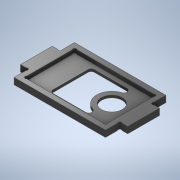
# Autodesk Inventor part: Trunk_servo_bottom_frame
Saved by Autodesk Inventor 2022 (Build 260153000, 153)
## iProperties
Part Number: Trunk_servo_bottom_frame
Material: アルミニウム 2014-T4
Document SubType Name: Sheet Metal
Designer: Masato Kubotera
Density: 2.8 g/cm^3
Appearance: 光沢 - 黒
Mass: 11.2606 g
Surface Area: 63.2089 cm^2
Volume: 7.90215 cm^3
Description: A2017 T4
Sheet Metal Rule: Default
Author: Masato Kubotera
Autodesk Inventor part; units mm, degrees
ref_plane "YZ Plane" through (0, 0, 0) normal (1, 0, 0) x (0, 1, 0)
ref_plane "XZ Plane" through (0, 0, 0) normal (0, 1, 0) x (-1, 0, 0)
ref_plane "XY Plane" through (0, 0, 0) normal (0, 0, 1) x (1, 0, 0)
sketch "スケッチ1" plane through (0, 0, 0) normal (0, 0, 1) x (1, 0, 0)
  line L0 (12, 16) -> (-29, 16) construction
  line L1 (-31, 14) -> (-31, -14) construction
  line L2 (-29, -16) -> (12, -16) construction
  line L3 (12, -16) -> (12, 16) construction
  line L4 (12, 16) -> (-31, -16) construction
  line L5 (-31, 16) -> (12, -16) construction
  line L6 (12, 0) -> (-31, 0) construction
  circle A0 centre (0, 0) radius 10.5 construction
  arc A1 (12, 10.583) -> (0, 16) centre (0, 0) ccw construction
  line L7 (-39.5, 14.4) -> (-39.5, -14.4) construction
  arc A2 (-29, 16) -> (-31, 14) centre (-29, 14) ccw construction
  arc A3 (-31, -14) -> (-29, -16) centre (-29, -14) ccw construction
  line L8 (-39.5, 14.4) -> (-30.9596, 14.4) construction
  line L9 (-39.5, -14.4) -> (-30.9596, -14.4) construction
  line L10 (-1, 13.5) -> (-28, 13.5) construction
  line L11 (-28, 13.5) -> (-28, -13.5) construction
  line L12 (-28, -13.5) -> (-1, -13.5) construction
  line L13 (-1, -13.5) -> (-1, 13.5) construction
  line L14 (-1, 13.5) -> (-28, -13.5) construction
  line L15 (-28, 13.5) -> (-1, -13.5) construction
  circle A4 centre (-1, 13.5) radius 1.35 construction
  circle A5 centre (-28, 13.5) radius 1.35 construction
  circle A6 centre (-1, -13.5) radius 1.35 construction
  circle A7 centre (-28, -13.5) radius 1.35 construction
  arc A8 (0, -16) -> (12, -10.583) centre (0, 0) ccw construction
  line L16 (11.9, 15.8) -> (11.9, 14.3151) construction
  line L17 (11.9, 15.8) -> (10.4151, 15.8) construction
  line L18 (-39.225, 15.8) -> (-39.225, 14.3151) construction
  arc A9 (-37.7401, 15.8) -> (-39.225, 14.3151) centre (-38.4825, 15.0575) ccw
  line L19 (11.9, -15.8) -> (10.4151, -15.8) construction
  arc A10 (-39.225, -14.3151) -> (-37.7401, -15.8) centre (-38.4825, -15.0575) ccw
  line L20 (-42.5, 19) -> (15, 19)
  line L21 (15, 19) -> (15, -19) construction
  line L22 (15, -19) -> (-42.5, -19)
  line L23 (-42.5, -19) -> (-42.5, 19) construction
  line L24 (-42.5, 19) -> (15, -19) construction
  line L25 (15, 19) -> (-42.5, -19) construction
  line L26 (15, 10) -> (16.4849, 10) construction
  line L27 (20, 10) -> (20, -10)
  line L28 (15, -10) -> (16.4849, -10) construction
  arc A11 (15, 11.4849) -> (16.4849, 10) centre (15.7425, 10.7425) ccw
  arc A12 (16.4849, -10) -> (15, -11.4849) centre (15.7425, -10.7425) ccw
  line L29 (-13.75, 19) -> (-13.75, -19) construction
  line L30 (15, 11.4849) -> (15, 19)
  line L31 (15, -11.4849) -> (15, -19)
  line L32 (-42.5, 10) -> (-43.9849, 10) construction
  line L33 (-47.5, 10) -> (-47.5, -10)
  line L34 (-42.5, -10) -> (-43.9849, -10) construction
  arc A13 (-43.9849, 10) -> (-42.5, 11.4849) centre (-43.2425, 10.7425) ccw
  arc A14 (-42.5, -11.4849) -> (-43.9849, -10) centre (-43.2425, -10.7425) ccw
  line L35 (-42.5, 11.4849) -> (-42.5, 19)
  line L36 (-42.5, -11.4849) -> (-42.5, -19)
  circle A15 centre (0, 0) radius 6 construction
  circle A16 centre (0, 0) radius 6.5
  line L37 (-3.5, 13) -> (-24, 13)
  line L38 (-26, 11) -> (-26, -11)
  line L39 (-3.5, -13) -> (-24, -13)
  arc A17 (-24, 13) -> (-26, 11) centre (-24, 11) ccw
  arc A18 (-26, -11) -> (-24, -13) centre (-24, -11) ccw
  line L40 (-1.5, 11) -> (-1.5, 10.9545)
  arc A19 (-2.8913, 9.0493) -> (-2.8913, -9.0493) centre (0, 0) ccw
  line L41 (-1.5, -10.9545) -> (-1.5, -11)
  arc A20 (-1.5, 11) -> (-3.5, 13) centre (-3.5, 11) ccw
  arc A21 (-3.5, -13) -> (-1.5, -11) centre (-3.5, -11) ccw
  arc A22 (-1.5, -10.9545) -> (-2.8913, -9.0493) centre (-3.5, -10.9545) ccw
  arc A23 (-2.8913, 9.0493) -> (-1.5, 10.9545) centre (-3.5, 10.9545) ccw
  arc A24 (11.9, 14.3151) -> (10.4151, 15.8) centre (11.1575, 15.0575) ccw
  arc A25 (10.4151, -15.8) -> (11.9, -14.3151) centre (11.1575, -15.0575) ccw
  line L42 (10.4151, 15.8) -> (-37.7401, 15.8)
  line L43 (11.9, 14.3151) -> (11.9, -14.3151)
  line L44 (10.4151, -15.8) -> (-37.7401, -15.8)
  line L45 (11.9, -14.3151) -> (11.9, -15.8) construction
  line L46 (-37.7401, -15.8) -> (-39.225, -15.8) construction
  line L47 (-39.225, -14.3151) -> (-39.225, -15.8) construction
  line L48 (-37.7401, 15.8) -> (-39.225, 15.8) construction
  line L49 (-39.225, 14.3151) -> (-39.225, -14.3151)
  line L50 (16.4849, 10) -> (20, 10)
  line L51 (16.4849, -10) -> (20, -10)
  line L52 (-43.9849, -10) -> (-47.5, -10)
  line L53 (-43.9849, 10) -> (-47.5, 10)
  point P0 (-9.5, 0)
  point P1 (-14.5, 0)
  point P2 (-13.75, 0)
  point P3 (-39.225, -14.3151)
  point P4 (-43.9849, -10)
  point P5 (-1.5, 13)
  point P6 (-26, 13)
  point P7 (-1.5, -13)
  point P8 (-26, -13)
  point P9 (-1.5, -13)
  point P10 (-1.5, 13)
  point P11 (-1.5, 9.3808)
  point P12 (-1.5, -9.3808)
  point P13 (11.9, -14.3151)
  point P14 (10.4151, -15.8)
  dimension "d0" = 43
  dimension "d1" = 32
  dimension "d2" = 21
  dimension "d3" = 16
  dimension "d4" = 9.5
  dimension "d5" = 28.8
  dimension "d7" = 2
  dimension "d8" = 8.5
  dimension "d9" = 27
  dimension "d10" = 27
  dimension "d11" = 8.5
  dimension "d12" = 2.7
  dimension "d13" = 2.7
  dimension "d23" = 3
  dimension "d24" = 3
  dimension "d26" = 5
  dimension "d27" = 20
  dimension "d29" = 1.05
  dimension "d34" = 12
  dimension "d35" = 13
  dimension "d36" = 38
  dimension "d39" = 5
  dimension "d40" = 2
  dimension "d43" = 3
  dimension "d44" = 3
  dimension "d45" = 1.5
  dimension "d46" = 2
  dimension "d47" = 2
  dimension "d54" = 51.125
  dimension "d55" = 0.1
  dimension "d57" = 31.6
  dimension "d58" = 2.1
  dimension "d59" = 2.1
  constraints: 108 end point, 44 point on circle, 30 symmetric about line, 26 centre point, 26 point on line, 17 tangent, 16 perpendicular, 10 horizontal, 10 midpoint, 8 coincident, 6 parallel, 4 collinear, 4 equal radius, 3 vertical, 1 concentric, 8 other
  measures "d0" distance of L2.end L4.end
  measures "d1" distance of L4.end L5.start
  measures "d2" diameter of A0
  measures "d3" radius of A1
  measures "d4" distance of point (-9.5, 0) A0.centre
  measures "d5" distance of L7.start L7.end
  measures "d7" radius of A2
  measures "d8" horizontal distance of L7.start L1.start
  measures "d9" distance of L12.end L11.end
  measures "d10" distance of L11.end L10.end
  measures "d11" horizontal distance of point (-9.5, 0) L10.start
  measures "d12" diameter of A4
  measures "d13" diameter of A5
  measures "d23" horizontal distance of L0.start L20.end
  measures "d24" horizontal distance of L7.start L20.start
  measures "d26" distance of L26.start L27.start
  measures "d27" distance of L27.start L27.end
  measures "d29" radius of A11
  measures "d34" diameter of A15
  measures "d35" diameter of A16
  measures "d36" distance of L21.end L20.end
  measures "d39" distance between parallel lines of L38 L1
  measures "d40" radius of A17
  measures "d43" radial gap between concentric circles of A19 A16
  measures "d44" distance between parallel lines of L37 L0
  measures "d45" horizontal distance of point (-1.5, 9.381) A0.centre
  measures "d46" radius of A20
  measures "d47" radius of A21
  measures "d54" distance from line of L16 L18.start
  measures "d55" distance between parallel lines of L16 L3
  measures "d57" distance between parallel lines of L19 L17
  measures "d58" diameter of A24
  measures "d59" diameter of A9
extrude "押し出し1" add sketch "スケッチ1" along normal blind 4 contours L20 L30 A11 L50 L27 L51 A12 L31 L22 L36 A14 L52 L33 L53 A13 L35
extrude "押し出し2" add sketch "スケッチ1" along normal blind 1.5 contours L42 A24 L43 A25 L44 A10 L49 A9
equation "\"d13\" = d12"
equation "\"d24\" = d23"
equation "\"d29\" = d17"
equation "\"d39\" = d38"
equation "\"d38\" = d37"
equation "\"d17\" = 1.05"
equation "\"d37\" = 5"
